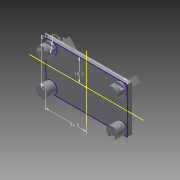
# Autodesk Inventor part: landframe
Saved by Autodesk Inventor 2015 (Build 190159000, 159)
## iProperties
Created: 2022-07-27
Part Number: landframe
Material: 常规
Document SubType Name: Modeling
Designer: Administrator
Density: 1 g/cm^3
Appearance: 默认
Author: Administrator
Autodesk Inventor part; units mm, degrees
ref_plane "YZ Plane" through (0, 0, 0) normal (1, 0, 0) x (0, 1, 0)
ref_plane "XZ Plane" through (0, 0, 0) normal (0, 1, 0) x (-1, 0, 0)
ref_plane "XY Plane" through (0, 0, 0) normal (0, 0, 1) x (1, 0, 0)
sketch "草图1" plane through (0, 0, 0) normal (0, 1, 0) x (-1, 0, 0)
  line L0 (34.5, 19.3) -> (-34.5, 19.3)
  line L1 (-34.5, 19.3) -> (-34.5, -19.3)
  line L2 (-34.5, -19.3) -> (34.5, -19.3)
  line L3 (34.5, -19.3) -> (34.5, 19.3)
  circle A0 centre (29.7, 14.5) radius 4.8
  line L4 (48.3, 0) -> (-48.3, 0) projected
  line L5 (0, -27.02) -> (0, 27.02) projected
  circle A1 centre (29.7, -14.5) radius 4.8
  circle A2 centre (-29.7, 14.5) radius 4.8
  circle A3 centre (-29.7, -14.5) radius 4.8
  point P0 (0, 0)
  dimension "d0" = 38.6
  dimension "d1" = 69
  dimension "d2" = 34.5
  dimension "d3" = 19.3
  dimension "d4" = 9.6
  constraints: 8 end point, 4 centre point, 3 symmetric about line, 2 parallel, 2 tangent, 1 horizontal, 1 perpendicular, 3 other
  measures "d0" distance of L2.end L0.start
  measures "d1" distance of L0.start L0.end
  measures "d2" distance from line of point (0, 0) L3
  measures "d3" distance from line of point (0, 0) L0
  measures "d4" diameter of A0
extrude "拉伸1" add sketch "草图1" along normal blind 4
extrude "拉伸2" add sketch "草图1" against normal blind 8 contours A0 | A2 | A1 | A3
sketch "草图2" plane through (0, 0, 0) normal (0, 0, 1) x (1, 0, 0)
  line L0 (24.9, -8) -> (34.5, -8) projected
  line L1 (34.5, 0) -> (29.7, 0) projected
  line L2 (29.7, 0) -> (34.5, 0) projected
  line L3 (34.5, 0) -> (34.5, -8) projected
  line L4 (34.5, -4.8) -> (32, -4.8)
  line L5 (32, -4.8) -> (32, -1.8)
  line L6 (32, -1.8) -> (34.5, -1.8)
  line L7 (34.5, -1.8) -> (34.5, -4.8)
  point P0 (0, 0)
  dimension "d9" = 1.8
  dimension "d10" = 3
  dimension "d11" = 2.5
  constraints: 8 end point, 2 parallel, 1 horizontal, 1 perpendicular, 1 point on line
  measures "d9" distance between parallel lines of L1 L6
  measures "d10" distance of L4.end L5.end
  measures "d11" distance of L4.start L4.end
extrude "拉伸3" [suppressed]
mirror "镜像1" [suppressed]
sketch "草图3" plane through (29.7, -8, -14.5) normal (0, -1, 0) x (1, 0, 0)
  arc A0 (2.3, -4.2131) -> (2.3, 4.2131) centre (0, 0) ccw projected
  circle A1 centre (0, 0) radius 4.8 projected
  line L0 (0, 0) -> (0, -4.8)
  line L1 (-2.5, -1.8) -> (2.5, -1.8)
  line L2 (2.5, -1.8) -> (2.5, -4.8)
  line L3 (2.5, -4.8) -> (-2.5, -4.8)
  line L4 (-2.5, -4.8) -> (-2.5, -1.8)
  line L5 (4.8, -4.8) -> (0, -4.8) projected
  point P0 (-29.7, 14.5)
  point P1 (2.4, -4.8)
  dimension "d17" = 2.5
  dimension "d18" = 5
  dimension "d19" = 3
  constraints: 10 end point, 2 parallel, 2 vertical, 1 horizontal, 1 midpoint, 1 perpendicular, 1 point on circle, 1 point on line, 1 vertical alignment
  measures "d17" distance between parallel lines of L0 L4
  measures "d18" distance of L1.start L1.end
  measures "d19" distance of L1.end L2.end
extrude "拉伸4" cut sketch "草图3" against normal through all contours L2 L3 A1 A0 | A0 A1 L0 L1 L2 | L4 L1 L0 A1 | A1 L3 L4
sketch "草图4" plane through (0, 4, 0) normal (0, 1, 0) x (1, 0, 0)
  line L0 (-48.3, 0) -> (48.3, 0) projected
  line L1 (0, 27.02) -> (0, -27.02) projected
  line L2 (28.3221, -16.1643) -> (19.8368, -7.679)
  line L3 (19.8368, -7.679) -> (23.3723, -4.1435)
  line L4 (23.3723, -4.1435) -> (31.8576, -12.6288)
  line L5 (31.8576, -12.6288) -> (28.3221, -16.1643)
  line L6 (34.5, -19.3) -> (17.3206, -2.1206)
  line L7 (-28.3221, -16.1643) -> (-19.8368, -7.679)
  line L8 (-19.8368, -7.679) -> (-23.3723, -4.1435)
  line L9 (-23.3723, -4.1435) -> (-31.8576, -12.6288)
  line L10 (-31.8576, -12.6288) -> (-28.3221, -16.1643)
  line L11 (28.3221, 16.1643) -> (19.8368, 7.679)
  line L12 (19.8368, 7.679) -> (23.3723, 4.1435)
  line L13 (23.3723, 4.1435) -> (31.8576, 12.6288)
  line L14 (31.8576, 12.6288) -> (28.3221, 16.1643)
  line L15 (-28.3221, 16.1643) -> (-19.8368, 7.679)
  line L16 (-23.3723, 4.1435) -> (-31.8576, 12.6288)
  line L17 (-31.8576, 12.6288) -> (-28.3221, 16.1643)
  line L18 (-19.8368, 7.679) -> (-23.3723, 4.1435)
  point P0 (0, 0)
  dimension "d22" = 5
  dimension "d23" = 12
  constraints: 34 end point, 12 symmetric about line, 2 parallel, 1 perpendicular, 1 other
  measures "d22" distance of L2.end L3.end
  measures "d23" distance of L2.start L2.end
extrude "拉伸5" add sketch "草图4" along normal blind 10
sketch "草图5" plane through (19.8368, 4, -7.679) normal (-0.7071, 0, -0.7071) x (-0.7071, 0, 0.7071)
  line L0 (0, 0) -> (-12, 0) projected
  line L1 (0, 0) -> (0, 10) projected
  line L2 (-12, 10) -> (0, 10) projected
  line L3 (-12, 0) -> (-12, 10) projected
  circle A0 centre (-6, 5) radius 1.5
  line L4 (-12, 10) -> (0, 10) projected
  line L5 (-6, 10) -> (-6, 0)
  point P0 (19.4566, -4)
  dimension "d26" = 3
  dimension "d27" = 5
  constraints: 3 midpoint, 2 end point, 1 centre point
  measures "d26" diameter of A0
  measures "d27" distance from line of L2 A0.centre
extrude "拉伸6" cut sketch "草图5" against normal blind 10 contours L5 A0 | A0 L5
mirror "镜像2" about plane through (0, 0, 0) normal (1, 0, 0) of "拉伸6"
mirror "镜像3" about plane through (0, 0, 0) normal (0, 0, 1) of "拉伸6"
mirror "镜像4" about plane through (0, 0, 0) normal (1, 0, 0) of "拉伸6", "镜像3"
sketch "草图6" plane through (0, 0, 0) normal (1, 0, 0) x (0, 1, 0)
  line L0 (-4.8, 16.8) -> (-1.8, 16.8)
  line L1 (-1.8, 16.8) -> (-1.8, 19.3)
  line L2 (-1.8, 19.3) -> (-4.8, 19.3)
  line L3 (-4.8, 19.3) -> (-4.8, 16.8)
  line L4 (0, 19.3) -> (-8.1735, 19.3)
  line L5 (0, 19.3) -> (0, 15.2583)
  point P0 (0, 0)
  point P1 (-3.3, 19.3)
  dimension "d30" = 3
  dimension "d31" = 2.5
  dimension "d32" = 1.8
  constraints: 12 end point, 2 horizontal, 2 parallel, 1 midpoint, 1 perpendicular, 1 point on line, 1 vertical
  measures "d30" distance of L0.start L0.end
  measures "d31" distance of L2.end L0.start
  measures "d32" distance between parallel lines of L5 L1
extrude "拉伸7" cut sketch "草图6" along normal through all both and the other way through all
mirror "镜像5" about plane through (0, 0, 0) normal (0, 0, 1) of "拉伸7"
